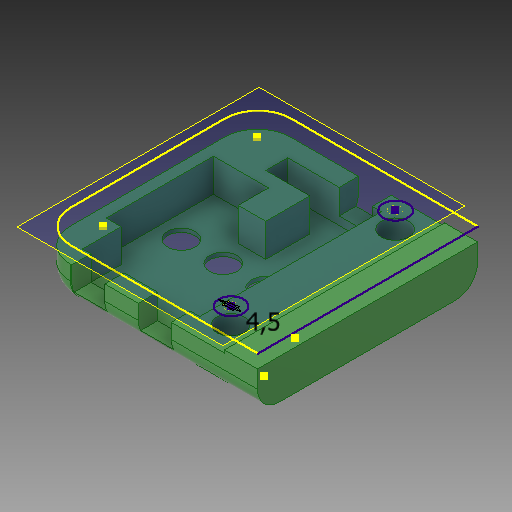
# Autodesk Inventor part: Holster_Top
Saved by Autodesk Inventor 2018 (Build 220112000, 112)
## iProperties
Created: 2018-02-02
Part Number: Holster_Top
Material: Generic
Document SubType Name: Modeling
Designer: Mandus
Density: 1 g/cm^3
Appearance: Smooth - Dark Forest Green
Author: Mandus
Autodesk Inventor part; units mm, degrees
ref_plane "YZ Plane" through (0, 0, 0) normal (1, 0, 0) x (0, 1, 0)
sketch "Sketch1" plane through (0, 0, 0) normal (0, 1, 0) x (-1, 0, 0)
  line L0 (7.1555, 5.751) -> (1.1555, 5.751)
  line L1 (1.1555, 5.751) -> (1.1555, -34.249)
  line L2 (1.1555, -34.249) -> (7.1555, -34.249)
  line L3 (7.1555, -34.249) -> (7.1555, 5.751)
  point P0 (0, 0)
  dimension "d0" = 6
  dimension "d1" = 40
  constraints: 8 end point, 2 parallel, 1 horizontal, 1 perpendicular
  measures "d0" distance of L2.end L1.end
  measures "d1" distance of L1.end L0.end
extrude "Extrusion1" add sketch "Sketch1" along normal blind 4
sketch "Sketch2" plane through (0, 0, 0) normal (0, -1, 0) x (1, 0, 0)
  line L0 (-1.1555, 5.751) -> (-1.1555, -34.249) projected
  line L1 (-1.1555, -34.249) -> (-41.1555, -34.249)
  line L2 (-41.1555, -34.249) -> (-41.1555, 5.751)
  line L3 (-41.1555, 5.751) -> (-1.1555, 5.751)
  line L4 (-1.1555, 5.751) -> (-1.1555, -34.249)
  circle A0 centre (-19.7555, -14.249) radius 2.5
  circle A1 centre (-27.3755, -14.249) radius 2.5
  circle A2 centre (-34.9955, -14.249) radius 2.5
  line L5 (-15.1555, -18.749) -> (-39.1555, -18.749)
  line L6 (-39.1555, -18.749) -> (-39.1555, -9.749)
  line L7 (-39.1555, -9.749) -> (-15.1555, -9.749)
  line L8 (-15.1555, -9.749) -> (-15.1555, -18.749)
  line L9 (-15.1555, -9.749) -> (-24.1555, -9.749)
  line L10 (-24.1555, -9.749) -> (-24.1555, 2.251)
  line L11 (-24.1555, 2.251) -> (-15.1555, 2.251)
  line L12 (-15.1555, 2.251) -> (-15.1555, -9.749)
  line L13 (-15.1555, -18.749) -> (-24.1555, -18.749)
  line L14 (-24.1555, -18.749) -> (-24.1555, -30.749)
  line L15 (-24.1555, -30.749) -> (-15.1555, -30.749)
  line L16 (-15.1555, -30.749) -> (-15.1555, -18.749)
  line L17 (-27.4555, -9.749) -> (-36.4555, -9.749)
  line L18 (-36.4555, -9.749) -> (-36.4555, 2.251)
  line L19 (-36.4555, 2.251) -> (-27.4555, 2.251)
  line L20 (-27.4555, 2.251) -> (-27.4555, -9.749)
  line L21 (-27.4555, 2.251) -> (-24.1555, 2.251)
  line L22 (-24.1555, -30.749) -> (-32.1555, -30.749)
  line L23 (-32.1555, -30.749) -> (-32.1555, -26.749)
  line L24 (-32.1555, -26.749) -> (-24.1555, -26.749)
  line L25 (-24.1555, -26.749) -> (-24.1555, -30.749)
  line L26 (-39.1555, -9.749) -> (-36.4555, -9.749)
  line L27 (-36.4555, -9.749) -> (-36.4555, -4.749)
  line L28 (-36.4555, -4.749) -> (-39.1555, -4.749)
  line L29 (-39.1555, -4.749) -> (-39.1555, -9.749)
  line L30 (-39.1555, -18.749) -> (-29.1555, -18.749)
  line L31 (-29.1555, -18.749) -> (-29.1555, -24.249)
  line L32 (-29.1555, -24.249) -> (-39.1555, -24.249)
  line L33 (-39.1555, -24.249) -> (-39.1555, -18.749)
  point P0 (0, 0)
  dimension "d4" = 40
  dimension "d5" = 40
  dimension "d6" = 5
  dimension "d7" = 20
  dimension "d8" = 21.4
  dimension "d9" = 2
  dimension "d10" = 9
  dimension "d11" = 4.5
  dimension "d12" = 24
  dimension "d13" = 7.62
  dimension "d14" = 7.62
  dimension "d15" = 9
  dimension "d16" = 12
  dimension "d17" = 9
  dimension "d18" = 12
  dimension "d19" = 9
  dimension "d20" = 12
  dimension "d21" = 3.3
  dimension "d61" = 8
  dimension "d62" = 4
  dimension "d63" = 2.7
  dimension "d64" = 5
  dimension "d65" = 10
  dimension "d66" = 5.5
  constraints: 66 end point, 16 parallel, 8 horizontal, 8 perpendicular, 3 centre point, 2 equal radius, 2 horizontal alignment, 1 point on line
  measures "d4" distance of L2.end L3.end
  measures "d5" distance of L1.end L2.end
  measures "d6" diameter of A0
  measures "d7" distance from line of L3 A0.centre
  measures "d8" distance from line of L2 A0.centre
  measures "d9" distance from line of L2 L6.end
  measures "d10" distance of L5.end L6.end
  measures "d11" vertical distance of A0.centre L7.end
  measures "d12" distance of L6.end L7.end
  measures "d13" distance of A1.centre A0.centre
  measures "d14" distance of A2.centre A1.centre
  measures "d15" distance of L10.end L11.end
  measures "d16" distance of L9.end L10.end
  measures "d17" distance of L15.end L14.end
  measures "d18" distance of L14.end L13.end
  measures "d19" distance of L18.end L19.end
  measures "d20" distance of L17.end L18.end
  measures "d21" distance from line of L20 L10.end
  measures "d61" distance of L23.end L24.end
  measures "d62" distance of L22.end L23.end
  measures "d63" distance of L28.end L27.end
  measures "d64" distance of L27.end L26.end
  measures "d65" distance of L31.end L32.end
  measures "d66" distance of L30.end L31.end
ref_plane "Work Plane1" through (-1.1555, -6.7, -3.7854) normal (0, -1, 0) x (1, 0, 0)
extrude "Extrusion2" add sketch "Sketch2" along normal up to surface (6.7 mm away) contours L0 L1 L2 L3 | L16 L15 L14 L5 | L5 L6 L7 L8 | L7 L10 L11 L12 | L31 L32 L33 L5 | L14 L22 L23 L24 | L7 L20 L21 L10 | L7 L18 L19 L20 | L29 L28 L18 L7
extrude "Extrusion3" cut sketch "Sketch2" along normal blind 6 contours L16 L15 L14 L5 | L5 L6 L7 L8 | L7 L10 L11 L12 | L31 L32 L33 L5 | L14 L22 L23 L24 | L7 L20 L21 L10 | L7 L18 L19 L20 | L29 L28 L18 L7
sketch "Sketch3" plane through (-7.1555, 4, 5.751) normal (0, 0, 1) x (1, 0, 0)
  point P0 (7.1555, -4)
sketch "Sketch4" plane through (0, 0, 0) normal (0, 1, 0) x (1, 0, 0)
  line L0 (-22.8196, 25.34) -> (-16.8196, 25.34)
  line L1 (-16.8196, 25.34) -> (-16.8196, 35.34)
  line L2 (-16.8196, 35.34) -> (-22.8196, 35.34)
  line L3 (-22.8196, 35.34) -> (-22.8196, 25.34)
  line L4 (-22.8196, 25.34) -> (-16.8196, 35.34) construction
  line L5 (-16.8196, 25.34) -> (-22.8196, 35.34) construction
  line L6 (-22.8196, 2.749) -> (-16.8196, 2.749)
  line L7 (-16.8196, 2.749) -> (-16.8196, -7.251)
  line L8 (-16.8196, -7.251) -> (-22.8196, -7.251)
  line L9 (-22.8196, -7.251) -> (-22.8196, 2.749)
  line L10 (-22.8196, 2.749) -> (-16.8196, -7.251) construction
  line L11 (-16.8196, 2.749) -> (-22.8196, -7.251) construction
  line L12 (-34.9085, 2.749) -> (-28.9085, 2.749)
  line L13 (-28.9085, 2.749) -> (-28.9085, -7.251)
  line L14 (-28.9085, -7.251) -> (-34.9085, -7.251)
  line L15 (-34.9085, -7.251) -> (-34.9085, 2.749)
  line L16 (-34.9085, 2.749) -> (-28.9085, -7.251) construction
  line L17 (-28.9085, 2.749) -> (-34.9085, -7.251) construction
  point P0 (0, 0)
  point P1 (-19.8196, 30.34)
  point P2 (-24.1555, 30.749)
  point P3 (-19.8196, -2.251)
  point P4 (-31.9085, -2.251)
  point P5 (-19.8196, 30.34)
  point P6 (-19.8196, -2.251)
  point P7 (-19.8196, -2.251)
  point P8 (-31.9085, -2.251)
  dimension "d40" = 6
  dimension "d41" = 10
  dimension "d42" = 6
  dimension "d43" = 10
  dimension "d44" = 6
  dimension "d45" = 10
  constraints: 36 end point, 10 midpoint, 6 parallel, 3 horizontal, 3 perpendicular, 1 horizontal alignment, 1 vertical alignment
  measures "d40" distance of L2.end L1.end
  measures "d41" distance of L1.end L0.end
  measures "d42" distance of L7.end L8.end
  measures "d43" distance of L6.end L7.end
  measures "d44" distance of L13.end L14.end
  measures "d45" distance of L12.end L13.end
extrude "Extrusion4" cut sketch "Sketch4" against normal blind 4.5
ref_plane "Work Plane2" through (-41.1555, 0, -10.749) normal (0, -1, 0) x (1, 0, 0)
fillet "Fillet4" radius 6 2 edges at (-41.1555, -3.35, 5.751) (-41.1555, -3.35, -34.249)
fillet "Fillet5" radius 4 5 edges at (-39.3981, -6.7, 3.9937) (-41.1555, -6.7, -14.249) (-39.3981, -6.7, -32.4916) (-18.1555, -6.7, -34.249) (-18.1555, -6.7, 5.751)
sketch "Sketch7" plane through (-35.1555, -6.7, -30.249) normal (0, -1, 0) x (1, 0, 0)
  circle A0 centre (24.1053, 31) radius 1 projected
  circle A1 centre (24, 1) radius 1 projected
  circle A2 centre (24.1053, 31) radius 2.5
  circle A3 centre (24, 1) radius 2.5
  point P0 (35.1555, 30.249)
  dimension "d70" = 5
  constraints: 2 centre point, 2 concentric, 1 equal radius
  measures "d70" diameter of A2
extrude "Extrusion6" cut sketch "Sketch7" against normal up to next contours A0 | A1 | A2 | A3
chamfer "Chamfer3" distance 2 angle 45 6 edges at (-8.7082, -6.7, -29.7597) (-11.6663, -6.7, -26.8017) (-11.1555, -6.4081, -31.749) (-11.561, -6.7, -1.6962) (-8.603, -6.7, 1.2618) (-11.0502, -6.4081, 3.251)
move faces "Move4" translate (0, -3.5, 0) faces at (-3.1555, 4, -7.5823)
ref_plane "Work Plane3" through (-40.3935, 3, -10.749) normal (0, -1, 0) x (-1, 0, 0)
sketch "Sketch8" plane through (-40.3935, 3, -10.749) normal (0, -1, 0) x (-1, 0, 0)
  arc A0 (-5.238, -16.5) -> (0.762, -10.5) centre (-5.238, -10.5) ccw projected
  line L0 (-5.238, -16.5) -> (-33.238, -16.5) projected
  line L1 (0.762, -10.5) -> (0.762, 17.5) projected
  arc A1 (0.762, 17.5) -> (-5.238, 23.5) centre (-5.238, 17.5) ccw projected
  line L2 (-5.238, 23.5) -> (-33.238, 23.5) projected
  line L3 (-39.238, 23.5) -> (-33.238, 23.5) projected
  line L4 (-39.238, -16.5) -> (-33.238, -16.5) projected
  line L5 (-39.238, -16.5) -> (-39.238, 23.5)
  circle A2 centre (-29.3433, -11.5) radius 1 construction
  circle A3 centre (-29.238, 18.5) radius 1 construction
  circle A4 centre (-29.3433, -11.5) radius 2.25
  circle A5 centre (-29.238, 18.5) radius 2.25
  point P0 (-40.3935, -10.749)
  dimension "d79" = 4.5
  constraints: 2 centre point, 2 coincident, 2 end point, 1 equal radius, 1 vertical
  measures "d79" diameter of A4
body "Solid1"
